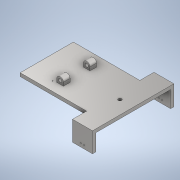
# Autodesk Inventor part: Steering Mount
Saved by Autodesk Inventor 2022 (Build 260153000, 153)
## iProperties
Created: 2021-12-07
Part Number: Steering Mount
Material: Generic
Document SubType Name: Sheet Metal
Designer: Vedic
Density: 1 g/cm^3
Appearance: Default
Sheet Metal Rule: Default
Author: Vedic
Autodesk Inventor part; units mm, degrees
ref_plane "YZ Plane" through (0, 0, 0) normal (1, 0, 0) x (0, 1, 0)
ref_plane "XZ Plane" through (0, 0, 0) normal (0, 1, 0) x (-1, 0, 0)
ref_plane "XY Plane" through (0, 0, 0) normal (0, 0, 1) x (1, 0, 0)
sketch "Sketch1" plane through (0, 0, 0) normal (0, 1, 0) x (-1, 0, 0)
  line L0 (111.0745, 206.7031) -> (-41.3255, 206.7031)
  line L1 (-41.3255, 206.7031) -> (-41.3255, -364.7969)
  line L2 (-41.3255, -364.7969) -> (111.0745, -364.7969)
  line L3 (111.0745, -364.7969) -> (111.0745, 206.7031)
  point P0 (0, 0)
  dimension "d0" = 571.5
  dimension "d1" = 152.4
  constraints: 8 end point, 2 parallel, 1 horizontal, 1 perpendicular
  measures "d0" distance of L2.end L0.start
  measures "d1" distance of L0.start L0.end
extrude "Extrusion1" add sketch "Sketch1" along normal blind 25.4
sketch "Sketch2" plane through (-111.0745, 0, 206.7031) normal (0, 0, 1) x (1, 0, 0)
  line L0 (0, 0) -> (0, 25.4) projected
  line L1 (0, 25.4) -> (152.4, 25.4)
  line L2 (152.4, 25.4) -> (152.4, -127)
  line L3 (152.4, -127) -> (0, -127)
  line L4 (0, -127) -> (0, 25.4)
  line L5 (152.4, 0) -> (152.4, 25.4) projected
  line L6 (0, 0) -> (152.4, 0) projected
  line L7 (0, -127) -> (152.4, -127)
  line L8 (152.4, -127) -> (152.4, -101.6)
  line L9 (152.4, -101.6) -> (0, -101.6)
  line L10 (0, -101.6) -> (0, -127)
  circle A0 centre (63.5, -101.6) radius 4.7625
  circle A1 centre (88.9, -101.6) radius 4.7625
  line L11 (0, -127) -> (63.5, -101.6) construction
  line L12 (88.9, -101.6) -> (152.4, -127) construction
  point P0 (111.0745, 0)
  point P1 (58.7375, -101.6)
  point P2 (68.2625, -101.6)
  point P3 (84.1375, -101.6)
  point P4 (93.6625, -101.6)
  dimension "d5" = 127
  dimension "d6" = 25.4
  dimension "d7" = 25.4
  dimension "d8" = 9.525
  constraints: 20 end point, 4 parallel, 3 point on line, 2 centre point, 2 horizontal, 2 perpendicular, 1 equal length, 1 equal radius
  measures "d5" distance between parallel lines of L3 L6
  measures "d6" distance between parallel lines of L9 L3
  measures "d7" distance of L12.start L11.end
  measures "d8" diameter of A1
extrude "Extrusion2" add sketch "Sketch2" along normal blind 25.4 contours L6 L2 L9 A1 A0 L4 | L0 L1 L2 L6 | L9 A0 A1 L2 L3 L4
sketch "Sketch3" plane through (41.3255, 0, -364.7969) normal (0, 0, -1) x (-1, 0, 0)
  line L0 (0, 25.4) -> (152.4, 25.4) projected
  line L1 (152.4, 0) -> (152.4, -127) projected
  line L2 (0, 25.4) -> (152.4, 25.4)
  line L3 (152.4, 25.4) -> (152.4, -127)
  line L4 (152.4, -127) -> (0, -127)
  line L5 (0, -127) -> (0, 25.4)
  circle A0 centre (63.5, -101.6) radius 4.7625 projected
  circle A1 centre (63.5, -101.6) radius 4.7625
  circle A2 centre (88.9, -101.6) radius 4.7625 projected
  circle A3 centre (88.9, -101.6) radius 4.7625
  point P0 (41.3255, 0)
  dimension "d15" = 9.525
  dimension "d16" = 9.525
  constraints: 8 end point, 2 centre point, 2 coincident, 2 parallel, 1 horizontal, 1 perpendicular
  measures "d15" diameter of A0
  measures "d16" diameter of A2
extrude "Extrusion3" add sketch "Sketch3" along normal blind 25.4
sketch "Sketch4" plane through (0, 25.4, 0) normal (0, 1, 0) x (1, 0, 0)
  line L0 (-52.337, 390.1969) -> (-42.812, 390.1969) construction
  line L1 (41.3255, -232.1031) -> (-111.0745, -232.1031) construction
  line L2 (-111.0745, -232.1031) -> (-111.0745, 390.1969) construction
  line L3 (-111.0745, 79.0469) -> (41.3255, 79.0469) construction
  line L4 (41.3255, 390.1969) -> (41.3255, -232.1031) construction
  line L5 (41.3255, 390.1969) -> (-111.0745, 390.1969) construction
  circle A0 centre (-60.2745, 79.0469) radius 12.7
  point P0 (0, 0)
  dimension "d17" = 25.4
  dimension "d20" = 50.8
  constraints: 2 end point, 2 midpoint, 1 centre point
  measures "d17" diameter of A0
  measures "d20" distance from line of L2 A0.centre
extrude "Extrusion4" cut sketch "Sketch4" against normal through all
sketch "Sketch5" plane through (0, 25.4, 0) normal (0, 1, 0) x (1, 0, 0)
  line L0 (-111.0745, -232.1031) -> (-111.0745, 390.1969) projected
  line L1 (-111.0745, 282.2469) -> (-619.0745, 282.2469)
  line L2 (-619.0745, 282.2469) -> (-619.0745, -124.1531)
  line L3 (-619.0745, -124.1531) -> (-111.0745, -124.1531)
  line L4 (-111.0745, -124.1531) -> (-111.0745, 282.2469)
  line L5 (41.3255, 390.1969) -> (-111.0745, 390.1969) construction
  line L6 (-619.0745, 282.2469) -> (-111.0745, 390.1969) construction
  line L7 (-111.0745, -232.1031) -> (-619.0745, -124.1531) construction
  point P0 (0, 0)
  point P1 (-111.0745, -124.1531)
  dimension "d21" = 508
  dimension "d22" = 406.4
  constraints: 12 end point, 2 parallel, 1 equal length, 1 horizontal, 1 perpendicular, 1 point on line
  measures "d21" distance of L2.end L3.end
  measures "d22" distance of L1.end L2.end
extrude "Extrusion5" add sketch "Sketch5" against normal blind 25.4
sketch "Sketch6" plane through (0, 25.4, 0) normal (0, 1, 0) x (1, 0, 0)
  line L0 (-619.0745, -124.1531) -> (-619.0745, 282.2469) construction
  line L1 (-619.0745, 282.2469) -> (-441.2745, 282.2469) construction
  line L2 (-441.2745, 282.2469) -> (-441.2745, -124.1531) construction
  line L3 (-441.2745, -124.1531) -> (-619.0745, -124.1531) construction
  line L4 (-619.0745, -124.1531) -> (-619.0745, 282.2469) construction
  circle A0 centre (-441.2745, 212.3969) radius 3.175
  circle A1 centre (-441.2745, -54.3031) radius 3.175
  line L5 (-619.0745, -124.1531) -> (-111.0745, -124.1531) projected
  line L6 (-111.0745, 282.2469) -> (-619.0745, 282.2469) projected
  line L7 (-111.0745, -232.1031) -> (-111.0745, -124.1531) projected
  line L8 (-111.0745, 282.2469) -> (-111.0745, 390.1969) projected
  point P0 (0, 0)
  dimension "d26" = 69.85
  dimension "d27" = 69.85
  dimension "d28" = 6.35
  dimension "d33" = 330.2
  dimension "d34" = 330.2
  constraints: 8 end point, 2 centre point, 2 parallel, 2 point on line, 1 equal radius, 1 horizontal, 1 perpendicular
  measures "d26" distance from line of L5 A1.centre
  measures "d27" distance from line of L6 A0.centre
  measures "d28" diameter of A0
  measures "d33" distance from line of L7 A1.centre
  measures "d34" distance from line of L8 A0.centre
extrude "Extrusion6" cut sketch "Sketch6" against normal through all
sketch "Sketch7" plane through (0, 25.4, 0) normal (0, 1, 0) x (1, 0, 0)
  line L0 (41.3255, -206.7031) -> (41.3255, 364.7969) construction
  line L1 (41.3255, 364.7969) -> (-365.0745, 364.7969) construction
  line L2 (-365.0745, 364.7969) -> (-365.0745, -206.7031) construction
  line L3 (-365.0745, -206.7031) -> (41.3255, -206.7031) construction
  line L4 (41.3255, -206.7031) -> (41.3255, 364.7969) construction
  line L5 (-619.0745, 282.2469) -> (-111.0745, 282.2469) construction
  line L6 (-365.0745, 282.2469) -> (-415.8745, 282.2469) construction
  line L7 (-415.8745, 282.2469) -> (-415.8745, -124.1531) construction
  line L8 (-415.8745, -124.1531) -> (-365.0745, -124.1531) construction
  line L9 (-365.0745, -124.1531) -> (-365.0745, 282.2469) construction
  line L10 (-415.8745, 282.2469) -> (-365.0745, 282.2469) construction
  line L11 (-365.0745, 282.2469) -> (-365.0745, -124.1531) construction
  line L12 (-365.0745, -124.1531) -> (-415.8745, -124.1531) construction
  line L13 (-415.8745, -124.1531) -> (-415.8745, 282.2469) construction
  line L14 (-415.8745, 206.0469) -> (-365.0745, 206.0469)
  line L15 (-365.0745, 206.0469) -> (-365.0745, 155.2469)
  line L16 (-365.0745, 155.2469) -> (-415.8745, 155.2469)
  line L17 (-415.8745, 155.2469) -> (-415.8745, 206.0469)
  line L18 (-415.8745, -47.9531) -> (-365.0745, -47.9531)
  line L19 (-365.0745, -47.9531) -> (-365.0745, 2.8469)
  line L20 (-365.0745, 2.8469) -> (-415.8745, 2.8469)
  line L21 (-415.8745, 2.8469) -> (-415.8745, -47.9531)
  point P0 (0, 0)
  dimension "d31" = 406.4
  dimension "d35" = 406.4
  dimension "d36" = 50.8
  dimension "d39" = 152.4
  dimension "d40" = 50.8
  dimension "d41" = 50.8
  dimension "d42" = 76.2
  dimension "d43" = 76.2
  constraints: 40 end point, 10 parallel, 5 horizontal, 5 perpendicular, 5 point on line, 1 midpoint
  measures "d31" distance of L0.start L2.end
  measures "d35" distance of L6.end L7.end
  measures "d36" distance between parallel lines of L2 L7
  measures "d39" distance between parallel lines of L16 L20
  measures "d40" distance between parallel lines of L16 L14
  measures "d41" distance between parallel lines of L20 L18
  measures "d42" distance between parallel lines of L12 L18
  measures "d43" distance between parallel lines of L5 L14
extrude "Extrusion7" add sketch "Sketch7" along normal blind 50.8
sketch "Sketch9" plane through (-415.8745, 25.4, 47.9531) normal (0, 0, 1) x (1, 0, 0)
  line L0 (50.8, 0) -> (50.8, 50.8) construction
  line L1 (50.8, 50.8) -> (0, 50.8) construction
  line L2 (50.8, 25.4) -> (25.4, 25.4) construction
  line L3 (25.4, 25.4) -> (25.4, 50.8) construction
  line L4 (25.4, 50.8) -> (50.8, 50.8) construction
  line L5 (50.8, 50.8) -> (50.8, 25.4) construction
  circle A0 centre (25.4, 25.4) radius 12.7
  point P0 (415.8745, -25.4)
  dimension "d44" = 25.4
  constraints: 8 end point, 2 midpoint, 2 parallel, 1 centre point, 1 coincident, 1 horizontal, 1 perpendicular
  measures "d44" diameter of A0
extrude "Extrusion8" cut sketch "Sketch9" against normal through all
fillet "Fillet1" radius 25.4 4 edges at (-415.8745, 76.2, 22.5531) (-365.0745, 76.2, 22.5531) (-415.8745, 76.2, -180.6469) (-365.0745, 76.2, -180.6469)
equation "\"d27\" = d26"
equation "\"BendRadius\" = Thickness"
equation "\"BendReliefWidth\" = Thickness"
equation "\"BendReliefDepth\" = 0.5 * Thickness"
equation "\"CornerReliefSize\" = 4 * Thickness"
equation "\"MinimumRemnant\" = 2 * Thickness"
equation "\"TransitionRadius\" = BendRadius"
equation "\"JacobiRadiusSize\" = BendRadius"
equation "\"GapSize\" = Thickness"
equation "\"Thickness\" = 3.048"
body "Solid1"
